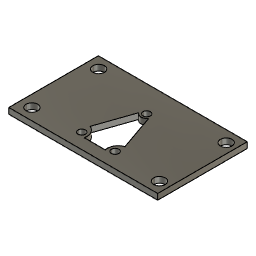
HeadFixer (Autodesk Fusion 360 design; units mm, degrees)
Autodesk Fusion 360 part; units mm, degrees
sketch "Sketch1" plane through (0, 0, 0) normal (0, 0, 1) x (1, 0, 0)
  line L0 (-28.5903, -0.0704) -> (11.5163, -0.0704)
  line L1 (11.5163, -0.0704) -> (11.5163, 24.0596)
  line L2 (11.5163, 24.0596) -> (-28.5903, 24.0596)
  line L3 (-28.5903, 24.0596) -> (-28.5903, -0.0704)
  line L4 (-8.537, 24.0596) -> (-8.537, -0.0704) construction
  line L5 (-28.5903, 3.0284) -> (11.5163, 3.0284) construction
  circle A0 centre (-25.4661, 21.0116) radius 1.5621
  circle A1 centre (8.8908, 21.0116) radius 1.5621
  circle A2 centre (8.8908, 3.0366) radius 1.5621
  circle A3 centre (-25.4661, 3.0366) radius 1.5621
  line L6 (-25.4661, 21.0116) -> (-25.4661, 3.0366) construction
  line L7 (-25.4661, 3.0366) -> (8.8908, 3.0366) construction
  line L8 (8.8908, 3.0366) -> (8.8908, 21.0116) construction
  line L9 (8.8908, 21.0116) -> (-25.4661, 21.0116) construction
  line L10 (-17.572, 16.5219) -> (-0.0282, 16.5219) construction
  line L11 (-13.6343, 7.2364) -> (-11.3582, 3.0366) construction
  line L12 (-5.7345, 3.0366) -> (-3.185, 7.5867) construction
  circle A4 centre (-8.537, 17.0283) radius 0.9998
  circle A5 centre (-4.0328, 4.0283) radius 0.9998
  circle A6 centre (-13.0328, 4.0283) radius 0.9998
  line L13 (-9.4819, 17.355) -> (-13.9777, 4.355) construction
  line L14 (-7.5923, 17.3556) -> (-3.0881, 4.3556) construction
  line L15 (-9.77, 16.5219) -> (-13.2356, 6.5009)
  line L16 (-7.3035, 16.5219) -> (-3.8169, 6.459)
  line L17 (-11.3582, 3.0366) -> (-5.7345, 3.0366)
  arc A7 (-11.3582, 3.0366) -> (-13.2356, 6.5009) centre (-14.3377, 3.6627) ccw
  arc A8 (-3.8169, 6.459) -> (-5.7345, 3.0366) centre (-2.8758, 3.6832) ccw
  arc A9 (-9.8839, 16.1927) -> (-7.1785, 16.1614) centre (-8.5198, 17.1617) ccw
  point P0 (-13.2356, 6.5009)
  point P1 (-3.8169, 6.459)
  dimension "d1" = 40.1066
  dimension "d2" = 24.13
  dimension "d12" = 3.0988
  dimension "d15" = 3.1242
  dimension "d16" = 3.048
  dimension "d17" = 3.1242
  dimension "d25" = 13
  dimension "d26" = 9
  dimension "d27" = 13
  dimension "d28" = 4.4958
  dimension "d29" = 4.5042
  constraint horizontal L0
  constraint vertical L1
  constraint horizontal L2
  constraint vertical L3
  constraint midpoint L2 L4.start
  constraint midpoint L0 L4.end
  constraint coincident L3 L5.start
  constraint coincident L1 L5.end
  constraint perpendicular L1 L5
  constraint equal A0 A1
  constraint equal A0 A2
  constraint equal A0 A3
  constraint coincident A0.centre L6.start
  constraint coincident A3.centre L6.end
  constraint coincident A2.centre L7.end
  constraint coincident A1.centre L8.end
  constraint perpendicular L5 L8
  constraint parallel L2 L9
  constraint parallel L0 L7
  constraint parallel L3 L6
  constraint coincident L7 L11.end
  constraint coincident L7 L12.start
  constraint coincident L4 A4.centre
  constraint tangent L5 A6
  constraint tangent L5 A5
  constraint tangent L11 A6
  constraint tangent L12 A5
  constraint coincident A4 L13.start
  constraint coincident A6 L13.end
  constraint tangent A4 L13
  constraint tangent A6 L13
  constraint coincident A4 L14.start
  constraint coincident A5 L14.end
  constraint tangent A5 L14
  constraint tangent A4 L14
  constraint coincident L13 P0
  constraint coincident L11 P0
  constraint coincident L12 P1
  constraint coincident L14 P1
  constraint coincident L10 L15.start
  constraint coincident L13 L15.start
  constraint coincident P0 L15.end
  constraint coincident L14 L16.start
  constraint coincident L10 L16.start
  constraint coincident P1 L16.end
  constraint parallel L14 L16
  constraint coincident L16 A9.end
  constraint coincident L13 A9.start
  constraint parallel L9 L10
  measures "d1" distance of L0.start L0.end
  measures "d2" distance of L0.start L2.end
  measures "d12" distance of L0 L5
  measures "d15" diameter of A0
  measures "d16" distance of L2 A0.centre
  measures "d17" distance of L3 A0.centre
  measures "d25" vertical distance of A5.centre A4.centre
  measures "d26" distance of A6.centre A5.centre
  measures "d27" vertical distance of A6.centre A4.centre
  measures "d28" horizontal distance of A6.centre A4.centre
  measures "d29" horizontal distance of A5.centre A4.centre
extrude "Extrude1" add sketch "Sketch1" along normal blind 1.5748
